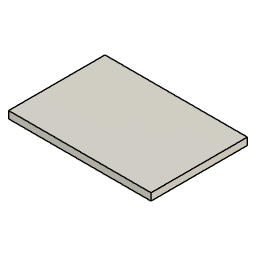
FinalExamBase v3 (Autodesk Fusion 360 design; units mm, degrees)
Autodesk Fusion 360 part; units mm, degrees
sketch "Sketch1" plane through (0, 0, 0) normal (0, 0, 1) x (1, 0, 0)
  line L0 (0, 0) -> (180, 0)
  line L1 (180, 0) -> (180, 65)
  line L2 (180, 65) -> (0, 65)
  line L3 (0, 65) -> (0, 0)
  dimension "d1" = 180
  dimension "d2" = 65
  constraint horizontal L0
  constraint vertical L1
  constraint horizontal L2
  constraint vertical L3
  constraint coincident L0.start L3.end
  measures "d1" distance of L0.start L0.end
  measures "d2" distance of L0.start L2.end
sketch "Sketch2" plane through (0, 0, 0) normal (0, 1, 0) x (1, 0, 0)
  line L0 (0, 0) -> (99, 0)
  line L1 (99, 0) -> (99, -67)
  line L2 (99, -67) -> (0, -67)
  line L3 (0, -67) -> (0, 0)
  dimension "d5" = 99
  dimension "d6" = 67
  constraint horizontal L0
  constraint vertical L1
  constraint horizontal L2
  constraint vertical L3
  constraint coincident L0.start L3.end
  measures "d5" distance of L0.start L0.end
  measures "d6" distance of L0.start L2.end
extrude "Extrude2" add sketch "Sketch2" along normal blind 5
move_body "Move1" bodies 1 to x (1, 0, 0) y (0, 0, -1) z (0, 1, 0) at (0, 5, 5)
